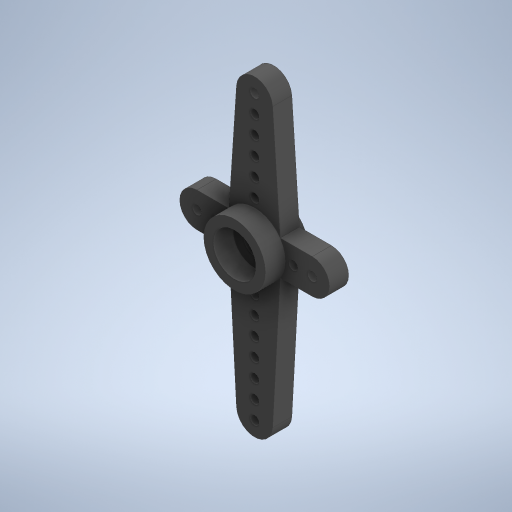
# Autodesk Inventor part: 180도 서보모터 십자축
Saved by Autodesk Inventor 2023.1 (Build 271208000, 208)
## iProperties
Created: 2021-08-22
Part Number: 180도 서보모터 십자축
Material: 일반
Document SubType Name: Modeling
Designer: fly01
Density: 1 g/cm^3
Appearance: 기본값
Author: fly01
Autodesk Inventor part; units mm, degrees
ref_plane "YZ Plane" through (0, 0, 0) normal (1, 0, 0) x (0, 1, 0)
ref_plane "XZ Plane" through (0, 0, 0) normal (0, 1, 0) x (-1, 0, 0)
ref_plane "XY Plane" through (0, 0, 0) normal (0, 0, 1) x (1, 0, 0)
sketch "스케치1" plane through (0, 0, 0) normal (0, 0, 1) x (1, 0, 0)
  circle A0 centre (0, 0) radius 2.5
  line L0 (-6.35, 0) -> (6.35, 0) construction
  line L1 (-6.35, -1.9) -> (6.35, -1.9)
  line L2 (6.35, 1.9) -> (-6.35, 1.9)
  arc A1 (-6.35, 1.9) -> (-6.35, -1.9) centre (-6.35, 0) ccw
  arc A2 (6.35, -1.9) -> (6.35, 1.9) centre (6.35, 0) ccw
  line L3 (0, 14.5) -> (0, -14.5) construction
  circle A3 centre (0, 14.5) radius 0.5
  circle A4 centre (0, -14.5) radius 0.5
  circle A5 centre (6.35, 0) radius 0.5
  circle A6 centre (-6.35, 0) radius 0.5
  circle A7 centre (-4.25, 0) radius 0.5
  circle A8 centre (4.25, 0) radius 0.5
  line L4 (0, -1.9) -> (0, -18.5)
  line L5 (0, 1.9) -> (0, 15.9)
  arc A9 (1.9954, 14.0355) -> (-1.9954, 14.0355) centre (0, 13.9) ccw
  arc A10 (-1.9969, -16.6117) -> (1.9969, -16.6117) centre (0, -16.5) ccw
  circle A11 centre (0, 0) radius 3.4
  line L6 (-1.9954, 14.0355) -> (-2.8196, 1.9)
  line L7 (1.9954, 14.0355) -> (2.8196, 1.9)
  line L8 (-2.8196, -1.9) -> (-1.9969, -16.6117)
  line L9 (2.8196, -1.9) -> (1.9969, -16.6117)
  circle A12 centre (0, 12.5) radius 0.5
  circle A13 centre (0, 10.5) radius 0.5
  circle A14 centre (0, 8.5) radius 0.5
  circle A15 centre (0, 6.5) radius 0.5
  circle A16 centre (0, 4.5) radius 0.5
  circle A17 centre (0, 0) radius 2.35
  circle A18 centre (0, -16.5) radius 0.5
  circle A19 centre (0, -12.5) radius 0.5
  circle A20 centre (0, -10.5) radius 0.5
  circle A21 centre (0, -8.5) radius 0.5
  circle A22 centre (0, -6.5) radius 0.5
  circle A23 centre (0, -4.5) radius 0.5
  dimension "d0" = 5
  dimension "d1" = 1.9
  dimension "d2" = 16.5
  dimension "d3" = 29
  dimension "d4" = 1
  dimension "d5" = 1
  dimension "d6" = 1
  dimension "d7" = 1
  dimension "d10" = 2.1
  dimension "d17" = 2.1
  dimension "d24" = 16.6
  dimension "d25" = 14
  dimension "d26" = 4
  dimension "d27" = 4
  dimension "d28" = 6.8
  dimension "d31" = 2
  dimension "d36" = 4.7
  dimension "d39" = 2
  dimension "d46" = 2
  constraints: 24 centre point, 22 end point, 14 point on circle, 10 point on line, 9 coincident, 8 tangent, 4 midpoint, 4 vertical, 3 horizontal, 1 parallel, 26 other
  measures "d0" diameter of A0
  measures "d1" radius of A2
  measures "d3" distance of L3.start L3.end
  measures "d4" diameter of A3
  measures "d5" diameter of A4
  measures "d6" diameter of A5
  measures "d7" diameter of A6
  measures "d10" distance of A6.centre A7.centre
  measures "d17" distance of A5.centre A8.centre
  measures "d24" distance of L4.start L4.end
  measures "d25" distance of L5.start L5.end
  measures "d26" diameter of A9
  measures "d27" diameter of A10
  measures "d28" diameter of A11
  measures "d31" distance of A3.centre A12.centre
  measures "d36" diameter of A17
  measures "d39" distance of A4.centre A18.centre
  measures "d46" distance of A4.centre A19.centre
extrude "돌출1" add sketch "스케치1" along normal blind 2.2 contours A0 L1 A17 L2 | A0 L2 A11 L1 | L2 A17 L5 A0 | A0 L5 A11 L2 | L1 A11 L4 A0 | A0 L4 A17 L1 | L5 A17 L2 A0 | A0 L2 A11 L5 | A17 L1 L2 | L2 L5 A17 | L4 A11 L1 A0 | A0 L1 A17 L4 | A17 L4 L1 | L2 A17 L1 A0 | A0 L1 A11 L2 | L5 L2 A17 | A17 L1 L4
extrude "돌출2" add sketch "스케치1" against normal blind 2.11 contours A0 L1 A17 L2 | A0 L2 A11 L1 | L2 A17 L5 A0 | A0 L5 A11 L2 | L1 A11 L4 A0 | A0 L4 A17 L1 | L5 A17 L2 A0 | A0 L2 A11 L5 | L2 A2 L1 A11 | A11 L5 A16 A15 A14 A13 A12 A3 A9 L7 | A17 L1 L2 | L2 L5 A17 | L4 A11 L1 A0 | A0 L1 A17 L4 | A17 L4 L1 | L9 A10 L4 A18 A4 A19 A20 A21 A22 A23 A11 | L2 A17 L1 A0 | A0 L1 A11 L2 | L5 L2 A17 | A11 L6 A9 L5 A3 A12 A13 A14 A15 A16 | A17 L1 L4 | L4 A23 A22 A21 A20 A19 A4 A18 A10 L8 A11 | A11 L1 A1 L2
extrude "돌출3" cut sketch "스케치1" along normal blind 3.65 contours A17 L1 L2 | L2 L5 A17 | A17 L4 L1 | L5 L2 A17 | A17 L1 L4
sketch "스케치2" plane through (0, 0, 0) normal (0, 0, 1) x (1, 0, 0)
  circle A0 centre (0, 0) radius 1.25
  dimension "d57" = 2.5
  constraints: 1 centre point, 1 coincident
  measures "d57" diameter of A0
extrude "돌출4" cut sketch "스케치2" against normal blind 7.6
sketch "스케치3" plane through (0, 0, -2.11) normal (0, 0, -1) x (-1, 0, 0)
  circle A0 centre (0, 0) radius 2.25
  dimension "d60" = 4.5
  constraints: 1 centre point, 1 coincident
  measures "d60" diameter of A0
extrude "돌출5" cut sketch "스케치3" against normal blind 1
sketch "스케치4" plane through (0, 0, -2.11) normal (0, 0, -1) x (-1, 0, 0)
  point P0 (0, 0)
sketch "스케치5" plane through (0, 0, -2.11) normal (0, 0, -1) x (-1, 0, 0)
  circle A0 centre (0, 0) radius 3.4
  circle A1 centre (0, 0) radius 2.25
  dimension "d63" = 4.5
  dimension "d64" = 6.8
  constraints: 2 centre point, 2 coincident
  measures "d63" diameter of A1
  measures "d64" diameter of A0
extrude "돌출6" add sketch "스케치5" along normal blind 0.4
sketch "스케치6" plane through (0, 0, -2.11) normal (0, 0, -1) x (-1, 0, 0)
  line L0 (0.9014, 15.3127) -> (-1.0592, 15.3127)
  line L1 (-1.0592, 15.3127) -> (-1.0592, 3.6394)
  line L2 (-1.0592, 3.6394) -> (0.9014, 3.6394)
  line L3 (0.9014, 3.6394) -> (0.9014, 15.3127)
  line L4 (1.0141, -3.7747) -> (-1.0592, -3.7747)
  line L5 (-1.0592, -3.7747) -> (-1.0592, -17.386)
  line L6 (-1.0592, -17.386) -> (1.0141, -17.386)
  line L7 (1.0141, -17.386) -> (1.0141, -3.7747)
  point P0 (0, 0)
  constraints: 16 end point, 4 parallel, 2 horizontal, 2 perpendicular, 1 point on line
extrude "돌출7" add sketch "스케치6" against normal blind 2.11
sketch "스케치7" plane through (0, 0, -2.11) normal (0, 0, -1) x (-1, 0, 0)
  circle A0 centre (0, 14.3) radius 0.5
  arc A1 (1.9954, 14.0355) -> (-1.9954, 14.0355) centre (0, 13.9) ccw projected
  line L0 (0, 0) -> (0, 0.7105)
  line L1 (0, 0) -> (0.8275, 0)
  circle A2 centre (0, 12.3) radius 0.5
  circle A3 centre (0, 10.3) radius 0.5
  circle A4 centre (0, 8.3) radius 0.5
  circle A5 centre (0, 6.3) radius 0.5
  circle A6 centre (0, 4.3) radius 0.5
  line L2 (0, 15.9) -> (3.4178, 15.9)
  arc A7 (1.9954, 14.0355) -> (-1.9954, 14.0355) centre (0, 13.9) ccw projected
  circle A8 centre (0, -16.9) radius 0.5
  arc A9 (-1.9969, -16.6117) -> (1.9969, -16.6117) centre (0, -16.5) ccw projected
  circle A10 centre (0, -14.9) radius 0.5
  circle A11 centre (0, -12.9) radius 0.5
  circle A12 centre (0, -10.9) radius 0.5
  circle A13 centre (0, -8.9) radius 0.5
  circle A14 centre (0, -6.9) radius 0.5
  circle A15 centre (0, -4.9) radius 0.5
  point P0 (0, -18.5)
  dimension "d69" = 1
  dimension "d73" = 2
  dimension "d78" = 1.6
  dimension "d79" = 1
  dimension "d80" = 1.6
  dimension "d86" = 2
  constraints: 13 centre point, 6 end point, 3 point on circle, 3 vertical, 2 horizontal, 1 tangent, 1 vertical alignment, 22 other
  measures "d69" diameter of A0
  measures "d73" distance of A0.centre A2.centre
  measures "d78" distance of A0.centre point (0, 15.9)
  measures "d79" diameter of A8
  measures "d80" distance of point (0, -18.5) A8.centre
  measures "d86" distance of A8.centre A10.centre
extrude "돌출8" cut sketch "스케치7" against normal blind 2.11
sketch "스케치9" plane through (0, 0, -2.11) normal (0, 0, -1) x (-1, 0, 0)
  circle A0 centre (0, 14.3) radius 0.5 projected
  circle A1 centre (0, -16.9) radius 0.5 projected
  point P0 (0, 0)
  dimension "d90" = 14.3
  dimension "d91" = 16.9
  measures "d90" distance of A0.centre point (0, 0)
  measures "d91" distance of A1.centre point (0, 0)
